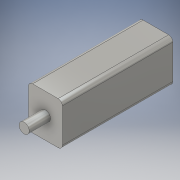
# Autodesk Inventor part: mtr
Saved by Autodesk Inventor 2016 (Build 200138000, 138)
## iProperties
Created: 2015-09-15
Part Number: mtr
Material: Generic
Document SubType Name: Modeling
Designer: cem
Density: 1 g/cm^3
Appearance: Default
Author: cem
Autodesk Inventor part; units mm, degrees
ref_plane "YZ Plane" through (0, 0, 0) normal (1, 0, 0) x (0, 1, 0)
ref_plane "XZ Plane" through (0, 0, 0) normal (0, 1, 0) x (-1, 0, 0)
ref_plane "XY Plane" through (0, 0, 0) normal (0, 0, 1) x (1, 0, 0)
sketch "Sketch1" plane through (0, 0, 0) normal (0, 1, 0) x (-1, 0, 0)
  line L0 (-5.08, 16.51) -> (5.08, 16.51)
  line L1 (5.08, 16.51) -> (5.08, -16.51)
  line L2 (5.08, -16.51) -> (-5.08, -16.51)
  line L3 (-5.08, -16.51) -> (-5.08, 16.51)
  line L4 (-5.08, 16.51) -> (5.08, -16.51) construction
  line L5 (5.08, 16.51) -> (-5.08, -16.51) construction
  point P0 (0, 0)
  dimension "d0" = 10.16
  dimension "d1" = 33.02
  constraints: 12 end point, 2 midpoint, 2 parallel, 1 horizontal, 1 perpendicular
  measures "d0" distance of L1.end L2.end
  measures "d1" distance of L0.end L1.end
extrude "Extrusion1" add sketch "Sketch1" along normal blind 12.7
fillet "Fillet1" radius 1.27 4 edges at (5.08, 12.7, 0) (5.08, 0, 0) (-5.08, 12.7, 0) (-5.08, 0, 0)
sketch "Sketch2" plane through (-3.81, 0, 16.51) normal (0, 0, 1) x (1, 0, 0)
  circle A0 centre (3.81, 6.35) radius 1.524
  point P0 (3.81, 0)
  dimension "d5" = 3.048
  constraints: 1 centre point
  measures "d5" diameter of A0
extrude "Extrusion2" add sketch "Sketch2" along normal blind 6.35
body "Solid1"
